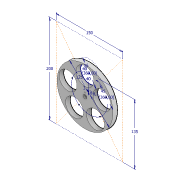
# Autodesk Inventor part: FilterWheel-M40-5pos
Saved by Autodesk Inventor 2021 (Build 250183000, 183)
## iProperties
Created: 2022-11-08
Part Number: FilterWheel-M40-5pos
Material: Generic
Document SubType Name: Modeling
Designer: nvladi
Density: 1 g/cm^3
Appearance: Default
Author: nvladi
Autodesk Inventor part; units mm, degrees
ref_plane "YZ Plane" through (0, 0, 0) normal (1, 0, 0) x (0, 1, 0)
ref_plane "XZ Plane" through (0, 0, 0) normal (0, 1, 0) x (-1, 0, 0)
ref_plane "XY Plane" through (0, 0, 0) normal (0, 0, 1) x (1, 0, 0)
sketch "Sketch1" plane through (0, 0, 0) normal (0, 0, 1) x (1, 0, 0)
  circle A0 centre (0, 0) radius 28 construction
  line L0 (75, -135) -> (-75, -135) construction
  line L1 (-75, -135) -> (-75, 65) construction
  line L2 (-75, 65) -> (75, 65) construction
  line L3 (75, 65) -> (75, -135) construction
  line L4 (75, -135) -> (-75, 65) construction
  line L5 (-75, -135) -> (75, 65) construction
  circle A1 centre (0, 0) radius 20
  circle A2 centre (-38.0423, -27.6393) radius 20
  circle A3 centre (-23.5114, -72.3607) radius 20
  circle A4 centre (23.5114, -72.3607) radius 20
  circle A5 centre (38.0423, -27.6393) radius 20
  circle A6 centre (0, -40) radius 62.5
  circle A7 centre (0, -40) radius 1.5
  circle A8 centre (0, -40) radius 4.05
  circle A9 centre (38.0423, -27.6393) radius 22.5 construction
  circle A10 centre (0, 0) radius 22.5 construction
  circle A11 centre (-38.0423, -27.6393) radius 22.5 construction
  circle A12 centre (-23.5114, -72.3607) radius 22.5 construction
  circle A13 centre (23.5114, -72.3607) radius 22.5 construction
  point P0 (0, -35)
  point P1 (0, -32)
  dimension "d0" = 56
  dimension "d1" = 150
  dimension "d2" = 200
  dimension "d3" = 135
  dimension "d4" = 40
  dimension "d7" = 360
  dimension "d9" = 40
  dimension "d10" = 125
  dimension "d11" = 3
  dimension "d12" = 8.1
  dimension "d17" = 45
  dimension "d20" = 360
  dimension "d22" = 8
  constraints: 14 centre point, 12 end point, 6 coincident, 2 midpoint, 2 parallel, 1 horizontal, 1 perpendicular, 22 other
  measures "d0" diameter of A0
  measures "d1" distance of L1.end L2.end
  measures "d2" distance of L0.end L1.end
  measures "d3" distance from line of L0 point (0, 0)
  measures "d4" diameter of A1
  measures "d9" distance of point (0, 0) point (0, -40)
  measures "d10" diameter of A6
  measures "d11" diameter of A7
  measures "d12" diameter of A8
  measures "d17" diameter of A9
  measures "d22" distance of point (0, -32) A6.centre
extrude "Extrusion1" add sketch "Sketch1" along normal blind 10 contours A6
extrude "Extrusion2" add sketch "Sketch1" along normal blind 7 contours A8
hole "Hole1" at (0, -40, 0) at (0, -32, 0) direction (0, 0, 1) diameter 2 end through all
body "Solid1"
